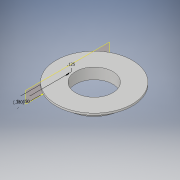
# Autodesk Inventor part: motor input
Saved by Autodesk Inventor 2019 (Build 230136000, 136)
## iProperties
Created: 2020-09-26
Part Number: motor input
Material: Generic
Document SubType Name: Modeling
Designer: Delta
Density: 1 g/cm^3
Appearance: Default
Author: Delta
Autodesk Inventor part; units mm, degrees
ref_plane "XZ Plane" through (0, 0, 0) normal (0, 1, 0) x (-1, 0, 0)
ref_plane "XY Plane" through (0, 0, 0) normal (0, 0, 1) x (1, 0, 0)
sketch "Sketch1" plane through (0, 0, 0) normal (0, 0, 1) x (1, 0, 0)
  line L0 (0, 0) -> (22.225, 0)
  line L1 (22.225, 7.62) -> (0, 7.62)
  line L2 (0, 7.62) -> (0, 0)
  line L3 (22.225, 9.144) -> (-9.525, 9.144)
  line L4 (-9.525, 9.144) -> (-9.525, 7.62)
  line L5 (22.225, 9.144) -> (22.225, 0)
  line L6 (-9.525, 7.62) -> (22.225, 7.62)
  dimension "d7" = 22.225
  constraints: 14 end point, 2 horizontal, 2 parallel, 1 perpendicular, 1 point on line
  measures "d7" distance between parallel lines of L2 L5
revolve "Revolution1" add sketch "Sketch1" angle 360 about axis through (22.225, 9.144, 0) along (0, -1, 0)
sketch "Sketch2" plane through (22.225, 9.144, 0) normal (0, 1, 0) x (1, 0, 0)
  circle A0 centre (0, 0) radius 31.75 projected
  circle A1 centre (0, 0) radius 15.494
  point P0 (-22.225, 0)
  dimension "d22" = 30.988
  constraints: 1 centre point, 1 coincident
  measures "d22" diameter of A1
extrude "Extrusion1" cut sketch "Sketch2" against normal through all contours A1
sketch "Sketch3" plane through (0, 0, 0) normal (1, 0, 0) x (0, 1, 0)
  line L0 (0, -22.225) -> (0, 22.225) projected
  line L1 (7.62, -22.225) -> (7.62, 22.225) projected
  circle A0 centre (3.81, 0) radius 1.5875
  point P0 (0, 0)
  dimension "d25" = 7.62
  dimension "d26" = 3.81
  dimension "d34" = 3.175
  constraints: 1 centre point, 1 coincident
  measures "d25" distance between parallel lines of L0 L1
  measures "d26" distance from line of L0 point (3.81, 0)
  measures "d34" diameter of A0
equation "\"d7\" = 0.5 * d1"
equation "\"d26\" = 0.5 * d25"
equation "\"d1\" = 44.45"
body "Solid1"
